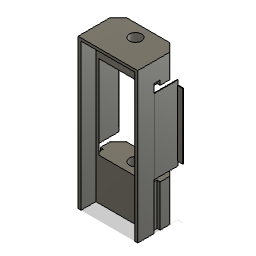
Optical_imaging_bed (Autodesk Fusion 360 design; units mm, degrees)
Autodesk Fusion 360 part; units mm, degrees
sketch "Sketch1" plane through (0, 0, 0) normal (0, 0, 1) x (1, 0, 0)
  line L0 (-20, 0) -> (20, 0)
  line L1 (20, 0) -> (20, 100)
  line L2 (20, 100) -> (-20, 100)
  line L3 (-20, 100) -> (-20, 0)
  line L4 (0, 0) -> (0, 160) construction
  dimension "d1" = 100
  dimension "d2" = 40
  constraint horizontal L0
  constraint vertical L1
  constraint horizontal L2
  constraint vertical L3
  constraint coincident L4.start origin
  constraint perpendicular L2 L4
  constraint symmetric L1 L3 L4
  measures "d1" distance of L0.start L2.end
  measures "d2" distance of L0.start L0.end
extrude "Extrude1" add sketch "Sketch1" along normal blind 14 and the other way blind 13 makes body 1
chamfer "Chamfer13" distance 5.5 angle 45 2 edges at (-20, 50, -13) (20, 50, -13) on bodies 1
sketch "Sketch2" plane through (0, 0, 14) normal (0, 0, 1) x (1, 0, 0)
  line L0 (-20, 100) -> (-20, 0)
  line L1 (-20, 0) -> (20, 0)
  line L2 (20, 0) -> (20, 100)
  line L3 (20, 100) -> (-20, 100)
  line L4 (-14.5, 0) -> (14.5, 0)
  line L5 (14.5, 0) -> (14.5, 100)
  line L6 (14.5, 100) -> (-14.5, 100)
  line L7 (-14.5, 100) -> (-14.5, 0)
  line L8 (0, 0) -> (0, 132.1606) construction
  line L9 (0, 0) -> (0, 70) construction
  dimension "d5" = 29
  constraint horizontal L4
  constraint vertical L5
  constraint horizontal L6
  constraint vertical L7
  constraint coincident L3 L5.end
  constraint coincident L1 L4.start
  constraint coincident L8.start L9.start
  constraint perpendicular L4 L8
  constraint symmetric L5 L7 L8
  constraint coincident L8 L9.end
  measures "d5" distance of L4.start L4.end
extrude "Extrude2" cut sketch "Sketch2" against normal blind 14 contours L1 L3 L4 L5 L6 L7 bodies 1
sketch "Sketch5" plane through (0, 0, 0) normal (0, 0, 1) x (1, 0, 0)
  line L0 (-14.5, 0) -> (14.5, 0)
  line L1 (14.5, 0) -> (14.5, 100)
  line L2 (14.5, 100) -> (-14.5, 100)
  line L3 (-14.5, 100) -> (-14.5, 0)
  line L4 (14.5, 93) -> (14.5, 86)
  line L5 (14.5, 86) -> (-14.5, 86)
  line L6 (-14.5, 86) -> (-14.5, 93)
  line L7 (-14.5, 0) -> (-14.5, 100)
  line L8 (14.5, 100) -> (14.5, 0)
  line L9 (-14.5, 93) -> (-8.2, 93)
  line L10 (-8.2, 86) -> (-14.5, 86)
  line L11 (-14.5, 86) -> (-14.5, 93)
  line L12 (14.5, 93) -> (8.2, 93)
  line L13 (14.5, 85.9926) -> (14.5, 93)
  line L14 (-14.5, 93) -> (-8.2, 93)
  line L15 (8.2, 93) -> (14.5, 93)
  point P0 (-5.5, 87)
  dimension "d32" = 7
  dimension "d33" = 86
  constraint horizontal L14
  constraint vertical L4
  constraint horizontal L5
  constraint vertical L6
  constraint collinear L3 L6
  constraint collinear L4 L8
  constraint horizontal L9
  constraint horizontal L10
  constraint vertical L11
  constraint horizontal L12
  constraint vertical L13
  constraint coincident L5 L10.start
  constraint collinear L14 L15
  measures "d32" distance of L6.end L5.end
  measures "d33" distance of origin L5
extrude "Extrude5" add sketch "Sketch5" along normal blind 4 bodies 1
ref_plane "WorkPlane1" through (0, 86, 0.5) normal (0, -1, 0) x (1, 0, 0)
move_face "OffsetFaces1" offset -3.5 1 faces at (-14.5, 66.6667, 10.6667) on bodies 1
move_face "OffsetFaces2" offset -3.5 1 faces at (14.5, 33.3333, 10.6667) on bodies 1
sketch "Sketch58" plane through (0, 0, 4) normal (0, 0, 1) x (1, 0, 0)
  line L0 (-18, 100) -> (-18, 0)
  line L1 (-18, 0) -> (18, 0)
  line L2 (18, 0) -> (18, 100)
  line L3 (-18, 100) -> (-18, 84) construction
  line L4 (-18, 84) -> (-16, 84) construction
  line L5 (-16, 84) -> (16, 84)
  line L6 (16, 84) -> (16, 28)
  line L7 (16, 28) -> (-16, 28)
  line L8 (-16, 28) -> (-16, 84)
  line L9 (18, 100) -> (-18, 100)
  dimension "d459" = 16
  dimension "d460" = 2
  dimension "d461" = 32
  dimension "d462" = 56
  constraint coincident L0.start L3.start
  constraint perpendicular L0 L4
  constraint horizontal L5
  constraint vertical L6
  constraint horizontal L7
  constraint vertical L8
  measures "d459" distance of L0.start L3.end
  measures "d460" distance of L3.end L4.end
  measures "d461" distance of L4.end L5.end
  measures "d462" distance of L4.end L7.end
extrude "Extrude83" cut sketch "Sketch58" against normal blind 30 contours L5 L6 L7 L8 bodies 1
sketch "Sketch59" plane through (0, 0, 0) normal (0, -1, 0) x (1, 0, 0)
  line L0 (20, -7.5) -> (20, 14)
  line L1 (20, 14) -> (18, 14)
  line L2 (18, 14) -> (18, 4)
  line L3 (18, 4) -> (-18, 4)
  line L4 (-18, 4) -> (-18, 14)
  line L5 (-18, 14) -> (-20, 14)
  line L6 (-20, 14) -> (-20, -7.5)
  line L7 (-14.5, -13) -> (14.5, -13)
  line L8 (0, 4) -> (0, -13) construction
  circle A0 centre (0, -4.5) radius 4.1
  line L9 (-20, 14) -> (-20, 1) construction
  line L10 (-20, 1) -> (-18, 1)
  line L11 (-18, 1) -> (-18, -1)
  line L12 (-18, -1) -> (-20, -1)
  line L13 (-20, -1) -> (-20, 1)
  line L14 (20, 1) -> (18, 1)
  line L15 (20, -1) -> (20, 1)
  line L16 (18, -1) -> (20, -1)
  line L17 (18, 1) -> (18, -1)
  line L18 (-20, -7.5) -> (-14.5, -13)
  line L19 (14.5, -13) -> (20, -7.5)
  dimension "d475" = 8.2
  dimension "d485" = 13
  dimension "d486" = 2
  dimension "d487" = 2
  constraint midpoint L3 L8.start
  constraint midpoint L7 L8.end
  constraint midpoint L8 A0.centre
  constraint coincident L5.end L6.start
  constraint perpendicular L5 L9
  constraint horizontal L10
  constraint vertical L11
  constraint horizontal L12
  constraint vertical L13
  constraint symmetric L8 L9.end L14.start
  constraint symmetric L8 L10.end L14.end
  constraint symmetric L8 L11.end L16.start
  constraint symmetric L8 L12.end L15.start
  measures "d475" diameter of A0
  measures "d485" distance of L5.end L9.end
  measures "d486" distance of L9.end L10.end
  measures "d487" distance of L9.end L12.end
extrude "Extrude84" cut sketch "Sketch59" against normal blind 100 contours A0 bodies 1
sketch "Sketch60" plane through (0, 0, -13) normal (0, 0, -1) x (-1, 0, 0)
  line L0 (-14.5, 84) -> (14.5, 84)
  line L1 (14.5, 28) -> (-14.5, 28)
  line L2 (14.5, 100) -> (-14.5, 100)
  line L3 (-14.5, 0) -> (14.5, 0)
  line L4 (0, 28) -> (0, 0) construction
  line L5 (0, 14) -> (20, 14) construction
  line L6 (0, 14) -> (0, 21) construction
  circle A0 centre (0, 21) radius 1.5
  circle A1 centre (0, 7) radius 1.5
  line L7 (-14.5, 28) -> (-14.5, 0)
  line L8 (14.5, 0) -> (14.5, 28)
  line L9 (14.5, 84) -> (14.5, 100)
  line L10 (-14.5, 100) -> (-14.5, 84)
  line L11 (0, 100) -> (0, 84) construction
  line L12 (-14.5, 92) -> (14.5, 92) construction
  circle A2 centre (0, 92) radius 1.5
  dimension "d478" = 3
  dimension "d512" = 3
  constraint midpoint L1 L4.start
  constraint coincident L4.end origin
  constraint midpoint L4 L5.start
  constraint coincident L4 L6.end
  constraint perpendicular L5 L6
  constraint coincident L6.end A0.centre
  constraint symmetric L5 A0 A1
  constraint midpoint L2 L11.start
  constraint midpoint L0 L11.end
  constraint midpoint L10 L12.start
  constraint midpoint L9 L12.end
  constraint midpoint L11 A2.centre
  measures "d478" diameter of A0
  measures "d512" diameter of A2
extrude "Extrude85" cut sketch "Sketch60" against normal blind 5 contours A0 | A1 | A2 bodies 1
extrude "Extrude86" cut sketch "Sketch59" against normal blind 87 contours L0 L14 L15 L16 L17 | L6 L10 L11 L12 L13 bodies 1
draft "Draft10" angle 45 neutral plane through (-18, 0, 1) pull (-1, 0, 0) 1 faces at (-19.3333, 29, 1) on bodies 1
draft "Draft11" angle 45 neutral plane through (18, 0, 1) pull (1, 0, 0) 1 faces at (19.3333, 29, 1) on bodies 1
draft "Draft8" angle -45 neutral plane through (0, 0, 4) pull (0, 0, 1) 1 faces at (16, 65.3333, -1.1667) on bodies 1
draft "Draft9" angle -45 neutral plane through (0, 0, 4) pull (0, 0, 1) 1 faces at (-16, 46.6667, -1.1667) on bodies 1
sketch "Sketch61" plane through (-20, 0, 0) normal (-1, 0, 0) x (0, 0, 1)
  line L0 (-7.5, 84) -> (-1, 84)
  line L1 (-1, 87) -> (3, 87)
  line L2 (3, 87) -> (3, 0)
  line L3 (3, 0) -> (14, 0)
  line L4 (14, 0) -> (14, 100)
  line L5 (3, 81.2319) -> (-13, 81.2319)
  line L6 (-13, 81.2319) -> (-13, 31.2319)
  line L7 (-13, 31.2319) -> (3, 31.2319)
  line L8 (3, 31.2319) -> (3, 81.2319)
  line L9 (14, 100) -> (-7.5, 100)
  line L10 (-7.5, 100) -> (-7.5, 84)
  line L11 (-1, 84) -> (-1, 87)
  dimension "d495" = 16
  dimension "d496" = 50
  constraint horizontal L5
  constraint vertical L6
  constraint horizontal L7
  constraint vertical L8
  constraint coincident L2 L5.start
  measures "d495" distance of L5.start L5.end
  measures "d496" distance of L5.start L7.end
extrude "Extrude87" add sketch "Sketch61" against normal blind 0.4 contours L2 L5 L6 L7 L8 bodies 1
sketch "Sketch62" plane through (20, 0, 0) normal (1, 0, 0) x (0, 0, -1)
  line L0 (1, 84) -> (7.5, 84)
  line L1 (-14, 100) -> (-14, 0)
  line L2 (-14, 0) -> (-3, 0)
  line L3 (-3, 0) -> (-3, 87)
  line L4 (-3, 87) -> (1, 87)
  line L5 (-3, 81.2319) -> (13, 81.2319)
  line L6 (13, 81.2319) -> (13, 31.2319)
  line L7 (13, 31.2319) -> (-3, 31.2319)
  line L8 (-3, 31.2319) -> (-3, 81.2319)
  line L9 (7.5, 100) -> (-14, 100)
  line L10 (7.5, 84) -> (7.5, 100)
  line L11 (1, 87) -> (1, 84)
  dimension "d499" = 16
  dimension "d500" = 50
  constraint horizontal L5
  constraint vertical L6
  constraint horizontal L7
  constraint vertical L8
  constraint coincident L3 L5.start
  measures "d499" distance of L5.start L5.end
  measures "d500" distance of L5.start L7.end
extrude "Extrude88" add sketch "Sketch62" against normal blind 0.4 contours L3 L5 L6 L7 L8 bodies 1
ref_plane "WorkPlane11" through (0, 50, 0.5) normal (1, 0, 0) x (0, 1, 0)
sketch "Sketch63" plane through (0, 0, -13) normal (0, 0, -1) x (-1, 0, 0)
  line L0 (-20, 81.2319) -> (-20, 31.2319)
  line L1 (-20, 31.2319) -> (-19.6, 31.2319)
  line L2 (-19.6, 31.2319) -> (-19.6, 81.2319)
  line L3 (-19.6, 81.2319) -> (-20, 81.2319)
  line L4 (-19.6, 81.2319) -> (-19.6, 78.2319) construction
  line L5 (-19.6, 78.2319) -> (-23.6, 78.2319)
  line L6 (-23.6, 78.2319) -> (-23.6, 34.2319)
  line L7 (-23.6, 34.2319) -> (-19.6, 34.2319)
  line L8 (-19.6, 34.2319) -> (-19.6, 78.2319)
  line L9 (0, -10) -> (0, 110)
  line L10 (19.6, 34.2319) -> (19.6, 78.2319)
  line L11 (19.6, 78.2319) -> (23.6, 78.2319)
  line L12 (23.6, 78.2319) -> (23.6, 34.2319)
  line L13 (23.6, 34.2319) -> (19.6, 34.2319)
  dimension "d505" = 3
  dimension "d506" = 4
  dimension "d507" = 44
  constraint coincident L2.end L3.start
  constraint perpendicular L3 L4
  constraint horizontal L5
  constraint vertical L6
  constraint horizontal L7
  constraint vertical L8
  constraint symmetric L4.end L9 L10.end
  constraint symmetric L5.end L9 L11.end
  constraint symmetric L6.end L9 L12.end
  constraint symmetric L7.end L9 L10.start
  measures "d505" distance of L2.end L4.end
  measures "d506" distance of L4.end L5.end
  measures "d507" distance of L4.end L7.end
extrude "Extrude89" add sketch "Sketch63" against normal blind 0.4 contours L0 L5 L6 L7 | L10 L11 L12 L13 bodies 1
sketch "Sketch1 (2)" plane through (0, 0, 0) normal (0, 1, 0) x (1, 0, 0) in component "Lid"
  line L0 (-20, -1.2) -> (-18.2, -1.2)
  line L1 (-18.2, -1.2) -> (-18.2, -2.8)
  line L2 (-18.2, -2.8) -> (-20, -2.8)
  line L3 (-20, -2.8) -> (-20.2, -2.8)
  line L4 (0, 0) -> (0, -35) construction
  line L5 (0, -35) -> (-30, -35) construction
  line L6 (0, -35) -> (0, -37) construction
  line L7 (0, -37) -> (-30, -37) construction
  line L8 (0, -35) -> (0, -37)
  line L9 (-20.2, -26.7415) -> (-22.2, -26.7415) construction
  line L10 (-22.2248, -1.2) -> (-20, -1.2)
  line L11 (0, -35) -> (0, -37)
  line L12 (22.2248, -1.2) -> (20, -1.2)
  line L13 (20, -1.2) -> (18.2, -1.2)
  line L14 (18.2, -1.2) -> (18.2, -2.8)
  line L15 (18.2, -2.8) -> (20, -2.8)
  line L16 (20, -2.8) -> (20.2, -2.8)
  line L17 (22.2248, -1.2) -> (-22.2248, -1.2)
  line L18 (-20.2, -2.8) -> (-20.2, -16)
  line L19 (-22.2248, -1.2) -> (-22.2248, -16)
  spline S0 degree 5 poles (-20.2, -16) (-20.2, -17.5712) (-19.9754, -20.5204) (-18.9656, -24.3653) (-16.4493, -28.4578) (-11.9406, -32.1721) (-7.568, -34.0819) (-3.927, -34.833) (-1.3362, -35) (0, -35) knots 0 0 0 0 0 0 0.2 0.4 0.6 0.8 1 1 1 1 1 1
  line L20 (-3, -35) -> (3, -35)
  line L21 (-20.2, -12.5385) -> (-20.2, -19.4615)
  spline S1 degree 5 poles (-22.2248, -16) (-22.2248, -17.57) (-22.0217, -20.5583) (-21.1083, -24.5853) (-18.7945, -29.1194) (-14.3577, -33.5036) (-9.567, -35.8565) (-5.143, -36.792) (-1.7829, -37) (0, -37) knots 0 0 0 0 0 0 0.2 0.4 0.6 0.8 1 1 1 1 1 1
  line L22 (-4, -37) -> (4, -37)
  line L23 (-22.2248, -12.5385) -> (-22.2248, -19.4615)
  spline S2 degree 5 poles (20.2, -16) (20.2, -17.5712) (19.9754, -20.5204) (18.9656, -24.3653) (16.4493, -28.4578) (11.9406, -32.1721) (7.568, -34.0819) (3.927, -34.833) (1.3362, -35) (0, -35) knots 0 0 0 0 0 0 0.2 0.4 0.6 0.8 1 1 1 1 1 1
  line L24 (20.2, -12.5385) -> (20.2, -19.4615)
  line L25 (3, -35) -> (-3, -35)
  spline S3 degree 5 poles (22.2248, -16) (22.2248, -17.57) (22.0217, -20.5583) (21.1083, -24.5853) (18.7945, -29.1194) (14.3577, -33.5036) (9.567, -35.8565) (5.143, -36.792) (1.7829, -37) (0, -37) knots 0 0 0 0 0 0 0.2 0.4 0.6 0.8 1 1 1 1 1 1
  line L26 (22.2248, -12.5385) -> (22.2248, -19.4615)
  line L27 (4, -37) -> (-4, -37)
  line L28 (22.2248, -1.2) -> (22.2248, -16)
  line L29 (20.2, -2.8) -> (20.2, -16)
  dimension "d402_1" = 35
  dimension "d403_1" = 2
  dimension "d404_1" = 30
  dimension "d405_1" = 2
  constraint horizontal L0
  constraint perpendicular L0 L1
  constraint perpendicular L1 L2
  constraint parallel L2 L3
  constraint coincident L4.start origin
  constraint vertical L4
  constraint perpendicular L4 L5
  constraint perpendicular L5 L6
  constraint perpendicular L6 L7
  constraint parallel L0 L10
  constraint symmetric L0.start L4 L12.end
  constraint symmetric L0.end L4 L13.end
  constraint symmetric L1.end L4 L14.end
  constraint symmetric L2.end L4 L15.end
  constraint symmetric L3.end L4 L16.end
  constraint symmetric L5.start L4 L6.start
  constraint symmetric L4 L6.end L7.start
  constraint symmetric L4 L10.start L12.start
  constraint horizontal L17
  constraint coincident L4.end L5.start
  constraint coincident L6.end L7.start
  constraint perpendicular L2 L18
  constraint perpendicular L17 L19
  constraint midpoint L4.end L20
  constraint midpoint L18.end L21
  constraint coincident L18 L21.start
  constraint midpoint L6.end L22
  constraint midpoint L19.end L23
  constraint coincident L19 L23.start
  constraint symmetric L4 L18.end S2.start
  constraint symmetric L4 L19.end S3.start
  constraint symmetric L4 L20.start L20.end
  constraint symmetric L4 L20.end L20.start
  constraint symmetric L4 L21.start L24.start
  constraint symmetric L4 L21.end L24.end
  constraint symmetric L4 L22.start L22.end
  constraint symmetric L4 L22.end L22.start
  constraint symmetric L4 L23.start L26.start
  constraint symmetric L4 L23.end L26.end
  measures "d402_1" distance of L4.start L4.end
  measures "d403_1" distance of L4.end L6.end
  measures "d404_1" distance of L6.end L7.end
  measures "d405_1" distance of L9.start L9.end
extrude "Extrude1'" add sketch "Sketch1 (2)" along normal blind 86.5 separate body contours L0 L1 L2 L3 L8 L10 L11 L17 L18 L19 S0 L21 S1 L23 | L8 L11 L12 L13 L14 L15 L16 L17 S2 L24 S3 L26 L28 L29 makes body 2 in component "Lid"
move_body "Move2" bodies 2 to x (1, 0, 0) y (0, 1, 0) z (0, 0, 1) at (-0.0863, 0, -1.8131) in component "Lid"
sketch "Sketch1 (3)" plane through (0, 0, 0) normal (0, 1, 0) x (1, 0, 0) in component "Lid (1)"
  line L0 (-20, -1.2) -> (-18.2, -1.2)
  line L1 (-18.2, -1.2) -> (-18.2, -2.8)
  line L2 (-18.2, -2.8) -> (-20, -2.8)
  line L3 (-20, -2.8) -> (-20.432, -2.8)
  line L4 (0, 0) -> (0, -28) construction
  line L5 (0, -28) -> (-30, -28) construction
  line L6 (0, -28) -> (0, -30) construction
  line L7 (0, -30) -> (-30, -30) construction
  line L8 (0, -28) -> (0, -30)
  line L9 (-20.2, -26.7415) -> (-22.2, -26.7415) construction
  line L10 (-22, -1.2) -> (-20, -1.2)
  line L11 (0, -28) -> (0, -30)
  line L12 (22, -1.2) -> (20, -1.2)
  line L13 (20, -1.2) -> (18.2, -1.2)
  line L14 (18.2, -1.2) -> (18.2, -2.8)
  line L15 (18.2, -2.8) -> (20, -2.8)
  line L16 (20, -2.8) -> (20.432, -2.8)
  line L17 (22, -1.2) -> (-22.2248, -1.2)
  line L18 (-20.432, -2.8) -> (-20.432, -13.3837)
  line L19 (-22, -1.2) -> (-22, -13.8454)
  spline S0 degree 5 poles (-20.432, -13.3837) (-20.432, -14.6806) (-20.1787, -17.0933) (-19.0394, -20.1691) (-16.2233, -23.3117) (-11.3507, -26.0211) (-6.9158, -27.3619) (-3.482, -27.8839) (-1.1652, -28) (0, -28) knots 0 0 0 0 0 0 0.2 0.4 0.6 0.8 1 1 1 1 1 1
  line L20 (-3, -28) -> (3, -28)
  line L21 (-20.432, -10.3643) -> (-20.432, -16.4031)
  spline S1 degree 5 poles (-22, -13.8454) (-22, -15.0661) (-21.7668, -17.3858) (-20.718, -20.5009) (-18.0949, -23.988) (-13.3197, -27.3391) (-8.5626, -29.1303) (-4.4892, -29.8418) (-1.536, -30) (0, -30) knots 0 0 0 0 0 0 0.2 0.4 0.6 0.8 1 1 1 1 1 1
  line L22 (-4, -30) -> (4, -30)
  line L23 (-22, -10.9493) -> (-22, -16.7415)
  spline S2 degree 5 poles (20.432, -13.3837) (20.432, -14.6806) (20.1787, -17.0933) (19.0394, -20.1691) (16.2233, -23.3117) (11.3507, -26.0211) (6.9158, -27.3619) (3.482, -27.8839) (1.1652, -28) (0, -28) knots 0 0 0 0 0 0 0.2 0.4 0.6 0.8 1 1 1 1 1 1
  line L24 (20.432, -10.3643) -> (20.432, -16.4031)
  line L25 (3, -28) -> (-3, -28)
  spline S3 degree 5 poles (22, -13.8454) (22, -15.0661) (21.7668, -17.3858) (20.718, -20.5009) (18.0949, -23.988) (13.3197, -27.3391) (8.5626, -29.1303) (4.4892, -29.8418) (1.536, -30) (0, -30) knots 0 0 0 0 0 0 0.2 0.4 0.6 0.8 1 1 1 1 1 1
  line L26 (22, -10.9493) -> (22, -16.7415)
  line L27 (4, -30) -> (-4, -30)
  line L28 (22, -1.2) -> (22, -13.8454)
  line L29 (20.432, -2.8) -> (20.432, -13.3837)
  dimension "d402_1_1" = 28
  dimension "d403_1_1" = 2
  dimension "d404_1_1" = 30
  dimension "d405_1_1" = 2
  constraint horizontal L0
  constraint perpendicular L0 L1
  constraint perpendicular L1 L2
  constraint parallel L2 L3
  constraint coincident L4.start origin
  constraint vertical L4
  constraint perpendicular L4 L5
  constraint perpendicular L5 L6
  constraint perpendicular L6 L7
  constraint parallel L0 L10
  constraint symmetric L0.start L4 L12.end
  constraint symmetric L0.end L4 L13.end
  constraint symmetric L1.end L4 L14.end
  constraint symmetric L2.end L4 L15.end
  constraint symmetric L3.end L4 L16.end
  constraint symmetric L5.start L4 L6.start
  constraint symmetric L4 L6.end L7.start
  constraint symmetric L4 L10.start L12.start
  constraint horizontal L17
  constraint coincident L4.end L5.start
  constraint coincident L6.end L7.start
  constraint perpendicular L2 L18
  constraint perpendicular L17 L19
  constraint midpoint L4.end L20
  constraint midpoint L18.end L21
  constraint coincident L18 L21.start
  constraint midpoint L6.end L22
  constraint midpoint L19.end L23
  constraint coincident L19 L23.start
  constraint symmetric L4 L18.end S2.start
  constraint symmetric L4 L19.end S3.start
  constraint symmetric L4 L20.start L20.end
  constraint symmetric L4 L20.end L20.start
  constraint symmetric L4 L21.start L24.start
  constraint symmetric L4 L21.end L24.end
  constraint symmetric L4 L22.start L22.end
  constraint symmetric L4 L22.end L22.start
  constraint symmetric L4 L23.start L26.start
  constraint symmetric L4 L23.end L26.end
  measures "d402_1_1" distance of L4.start L4.end
  measures "d403_1_1" distance of L4.end L6.end
  measures "d404_1_1" distance of L6.end L7.end
  measures "d405_1_1" distance of L9.start L9.end
extrude "Extrude1''" add sketch "Sketch1 (3)" along normal blind 86.5 separate body contours L0 L1 L2 L3 L8 L10 L11 L17 L18 L19 S0 L21 S1 L23 | L8 L11 L12 L13 L14 L15 L16 L17 S2 L24 S3 L26 L28 L29 makes body 3 in component "Lid (1)"
move_body "Move2'" bodies 3 to x (1, 0, 0) y (0, 1, 0) z (0, 0, 1) at (-0.0863, 0, -1.8131) in component "Lid (1)"
ref_plane "WorkPlane13" through (-19, 50, 14) normal (0, 0, 1) x (1, 0, 0)
ref_plane "WorkPlane14" through (0, 50, 14) normal (0, 0, 1) x (1, 0, 0)
sketch "Sketch64" plane through (0, 50, 14) normal (0, 0, 1) x (1, 0, 0)
  line L0 (-20, 50) -> (20, 50)
  line L1 (20, 50) -> (20, 40)
  line L2 (20, 40) -> (-20, 40)
  line L3 (-20, 40) -> (-20, 50)
  dimension "d515" = 40
  dimension "d516" = 10
  constraint horizontal L0
  constraint vertical L1
  constraint horizontal L2
  constraint vertical L3
  measures "d515" distance of L0.start L0.end
  measures "d516" distance of L0.start L2.end
sketch "Sketch65" plane through (18, 0, 0) normal (-1, 0, 0) x (0, 0, 1)
  line L0 (4, 100) -> (4, 0)
  line L1 (4, 0) -> (14, 0)
  line L2 (14, 0) -> (14, 100)
  line L3 (14, 100) -> (4, 100)
  line L4 (4, 100) -> (14, 100)
  line L5 (14, 100) -> (14, 98.2)
  line L6 (14, 98.2) -> (4, 98.2)
  line L7 (4, 98.2) -> (4, 100)
  dimension "d519" = 10
  dimension "d520" = 1.8
  constraint horizontal L4
  constraint vertical L5
  constraint horizontal L6
  constraint vertical L7
  constraint coincident L0.start L3.end
  measures "d519" distance of L0.start L2.end
  measures "d520" distance of L0.start L6.end
extrude "Extrude91" add sketch "Sketch65" along normal blind 36 contours L0 L2 L3 L4 L5 L6 L7 bodies 1
component "Lid" placed x (1, 0, 0) y (0, 1, 0) z (0, 0, 1) at (0, 0, 0)
component "Lid (1)" placed x (1, 0, 0) y (0, 1, 0) z (0, 0, 1) at (0, 0, 0)
